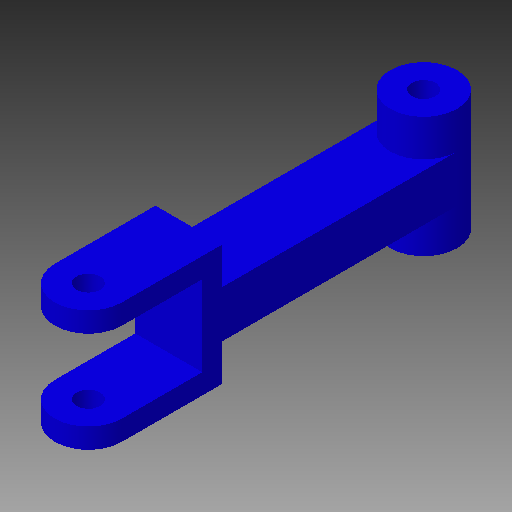
# Autodesk Inventor part: 筷子套軸
Saved by Autodesk Inventor 2017 (Build 210142000, 142)
## iProperties
Created: 2019-12-02
Part Number: 筷子套軸
Material: 一般
Document SubType Name: Modeling
Designer: 吳昇峻
Density: 1 g/cm^3
Appearance: 預設
Mass: 4.85354 g
Surface Area: 32.0357 cm^2
Volume: 4.85354 cm^3
Author: 吳昇峻
Autodesk Inventor part; units mm, degrees
ref_plane "YZ Plane" through (0, 0, 0) normal (1, 0, 0) x (0, 1, 0)
ref_plane "XY Plane" through (0, 0, 0) normal (0, 0, 1) x (1, 0, 0)
sketch "草圖1" plane through (0, 0, 0) normal (0, 1, 0) x (-1, 0, 0)
  circle A0 centre (0, 0) radius 1.75
  arc A1 (5, 0) -> (-5, 0) centre (0, 0) ccw
  circle A2 centre (0, -50) radius 1.75
  arc A3 (-5, -50) -> (5, -50) centre (0, -50) ccw
  line L0 (5, 0) -> (5, -50)
  line L1 (-5, 0) -> (-5, -50)
  dimension "d1" = 3.5
  dimension "d2" = 10
  dimension "d3" = 3.5
  dimension "d4" = 10
  dimension "d36" = 50
  constraints: 4 centre point, 4 end point, 4 point on circle, 3 coincident, 2 tangent
  measures "d1" diameter of A0
  measures "d2" diameter of A1
  measures "d3" diameter of A2
  measures "d4" diameter of A3
  measures "d36" distance of L1.end L1.start
extrude "擠出1" add sketch "草圖1" along normal blind 7
sketch "草圖2" plane through (0, 7, 0) normal (0, 1, 0) x (1, 0, 0)
  line L0 (0, 0) -> (0, 15) construction
  line L1 (-5, 50) -> (-5, 0) projected
  line L2 (5, 0) -> (5, 50) projected
  arc A0 (-5, 0) -> (5, 0) centre (0, 0) ccw projected
  circle A1 centre (0, 0) radius 1.75 projected
  line L3 (-5, 15) -> (5, 15)
  point P0 (-5, 9)
  point P1 (5, 9)
  dimension "d7" = 15
  constraints: 4 end point, 4 point on line, 1 perpendicular, 1 vertical
  measures "d7" distance of L0.start L0.end
sketch "草圖3" plane through (0, 0, 0) normal (0, -1, 0) x (1, 0, 0)
  line L0 (-5, -9) -> (5, -9) projected
  arc A0 (5, 0) -> (-5, 0) centre (0, 0) ccw projected
  line L1 (-5, -50) -> (-5, 0) projected
  circle A1 centre (0, 0) radius 1.75 projected
  line L2 (5, 0) -> (5, -50) projected
extrude "擠出2" add sketch "草圖2" along normal blind 5.5
sketch "草圖5" plane through (0, 7, 0) normal (0, 1, 0) x (1, 0, 0)
  circle A0 centre (0, 50) radius 1.75 projected
  circle A1 centre (0, 50) radius 5
  point P0 (0, 0)
  dimension "d17" = 10
  constraints: 1 centre point, 1 coincident
  measures "d17" diameter of A1
extrude "擠出5" add sketch "草圖5" along normal blind 5.5
sketch "草圖6" plane through (0, 0, 0) normal (0, -1, 0) x (1, 0, 0)
  circle A0 centre (0, -50) radius 1.75 projected
  circle A1 centre (0, -50) radius 5
  point P0 (0, 0)
  dimension "d20" = 10
  constraints: 1 centre point, 1 coincident
  measures "d20" diameter of A1
extrude "擠出6" add sketch "草圖6" along normal blind 5.5
sketch "草圖9" plane through (0, 0, 0) normal (0, -1, 0) x (1, 0, 0)
  circle A0 centre (0, 0) radius 1.75 projected
  circle A1 centre (0, 0) radius 1.75 projected
  line L0 (-5, -15) -> (-5, 0) projected
  arc A2 (5, 0) -> (-5, 0) centre (0, 0) ccw projected
  line L1 (5, 0) -> (5, -15) projected
  line L2 (5, -15) -> (-5, -15) projected
extrude "擠出7" add sketch "草圖9" along normal blind 5.5
sketch "草圖10" plane through (-5, 0, -50) normal (-1, 0, 0) x (0, 0, 1)
  line L0 (55, 12.5) -> (50, 12.5) construction
  line L1 (55, 12.5) -> (55, 9.5) construction
  line L2 (55, -5.5) -> (55, 12.5) construction
  line L3 (55, 9.5) -> (38, 9.5)
  line L4 (38, 9.5) -> (38, -2.5)
  line L5 (38, -2.5) -> (55, -2.5)
  line L6 (55, 9.5) -> (55, -2.5)
  point P0 (50, 0)
  dimension "d25" = 3
  dimension "d26" = 17
  dimension "d27" = 12
  constraints: 10 end point, 3 perpendicular, 2 point on line, 1 horizontal
  measures "d25" distance of L0.start L1.end
  measures "d26" distance of L1.end L3.end
  measures "d27" distance of L3.end L4.end
extrude "擠出8" cut sketch "草圖10" against normal up to next
ref_plane "工作平面1" through (0, 3.5, 0) normal (0, 1, 0) x (-1, 0, 0)
sketch "草圖11" plane through (0, 3.5, 0) normal (0, 1, 0) x (-1, 0, 0)
  circle A0 centre (0, 0) radius 1.75 projected
  line L0 (5, -15) -> (5, 0) projected
  arc A1 (5, 0) -> (-5, 0) centre (0, 0) ccw projected
  line L1 (-5, 0) -> (-5, -15) projected
  line L2 (-5, -15) -> (5, -15) projected
  arc A2 (5, -50) -> (-5, -50) centre (0, -50) ccw projected
  line L3 (5, -50) -> (5, -15) projected
  line L4 (5, -15) -> (-5, -15) projected
  line L5 (-5, -15) -> (-5, -50) projected
  circle A3 centre (0, -50) radius 1.75 projected
  circle A4 centre (0, -50) radius 5 projected
  dimension "d35" = 50
  measures "d35" distance of A2.centre point (0, 0)
